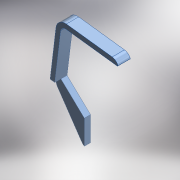
# Autodesk Inventor part: HousingArm0
Saved by Autodesk Inventor 2018 (Build 220112000, 112)
## iProperties
Created: 2019-04-09
Part Number: HousingArm0
Material: PLA Plastic (Glacial Blue)
Document SubType Name: Modeling
Designer: Isaac Newcomb
Density: 1.06 g/cm^3
Appearance: 3D Printed - Glacial Blue
Mass: 6.25093 g
Surface Area: 40.4006 cm^2
Volume: 5.8971 cm^3
d8: 15.000 mm
Author: Isaac Newcomb
Autodesk Inventor part; units mm, degrees
ref_plane "YZ Plane" through (0, 0, 0) normal (1, 0, 0) x (0, 1, 0)
ref_plane "XZ Plane" through (0, 0, 0) normal (0, 1, 0) x (-1, 0, 0)
ref_plane "XY Plane" through (0, 0, 0) normal (0, 0, 1) x (1, 0, 0)
sketch "Base Sketch" plane through (0, 0, 0) normal (0, 0, 1) x (1, 0, 0)
  line L0 (22, 0) -> (0, 0)
  line L1 (3.4939, 2.3817) -> (36.1282, 24.6282)
  line L2 (41, 20) -> (22, 0)
  line L3 (41, 20) -> (85.6646, 14.5159)
  line L4 (90.1222, 17.9986) -> (36.1282, 24.6282)
  line L5 (36.1282, 24.6282) -> (41, 20) construction
  line L6 (41, 20) -> (41.4875, 23.9702)
  line L7 (3.4939, 2.3817) -> (0, 0) construction
  line L8 (0, 0) -> (0, -2.6652) construction
  arc A0 (3.4939, 2.3817) -> (0, -4.2285) centre (8, -4.2285) ccw
  line L9 (85.6646, 14.5159) -> (79.693, -34.1189)
  line L10 (79.693, -34.1189) -> (83.6632, -34.6064)
  line L11 (83.6632, -34.6064) -> (90.1222, 17.9986)
  point P0 (1.2088, 0)
  dimension "d2" = 22
  dimension "d3" = 20
  dimension "d4" = 19
  dimension "d5" = 4
  dimension "d24" = 8
  dimension "d25" = 4
  dimension "d27" = 7
  dimension "d28" = 45
  dimension "d29" = 49
  constraints: 25 end point, 5 perpendicular, 3 point on circle, 3 point on line, 2 tangent, 1 centre point, 1 coincident, 1 collinear, 1 horizontal, 1 parallel, 1 vertical
  measures "d2" distance of L0.start L0.end
  measures "d3" distance from line of L0 L2.start
  measures "d4" horizontal distance of L2.start L0.start
  measures "d5" distance between parallel lines of L4 L3
  measures "d24" radius of A0
  measures "d25" distance between parallel lines of L11 L9
  measures "d27" angle of L0 L3
  measures "d28" distance of L2.start L3.end
  measures "d29" distance of L3.end L9.end
extrude "Lower Arm" add sketch "Base Sketch" along normal blind 5.25 contours L0 A0 L1 L4 L6 L2
extrude "Upper Arm" add sketch "Base Sketch" along normal blind 10.5 contours L6 L4 L11 L10 L9 L3
fillet "Fillet1" radius 8 2 edges at (36.1282, 24.6282, 2.625) (90.1222, 17.9986, 5.25)
fillet "Fillet1" radius 4 1 edges at (85.6646, 14.5159, 5.25)
fillet "Fillet3" radius 6 1 edges at (83.6632, -34.6064, 5.25)
fillet "Fillet4" radius 0.4 1 edges at (79.693, -34.1189, 5.25)
equation "\"d2\" = ConnectionWidth"
equation "\"d3\" = ArmDistance"
equation "\"d4\" = ArmTravelToDistance"
equation "\"d5\" = ArmThickness"
equation "\"d25\" = ArmThickness"
equation "\"d18\" = 0.5 * KeySpacing + 0.5 * KeyWidth"
equation "\"d20\" = KeyWidth + KeySpacing"
equation "\"ConnectionWidth\" = 22"
equation "\"ArmDistance\" = 20"
equation "\"ArmTravelToDistance\" = 19"
equation "\"ArmThickness\" = 4"
equation "\"KeySpacing\" = 0.5"
equation "\"KeyWidth\" = 10"
body "Solid2"
